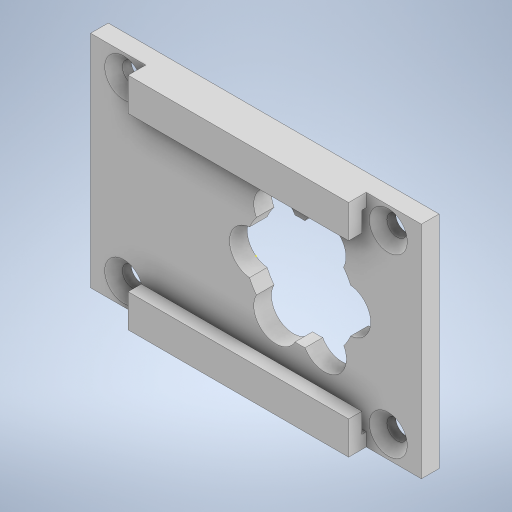
# Autodesk Inventor part: lid support
Saved by Autodesk Inventor 2023.3 (Build 273359000, 359)
## iProperties
Created: 2022-03-16
Part Number: lid support
Material: Generic
Document SubType Name: Modeling
Designer: sawtelles
Density: 1 g/cm^3
Appearance: Default
Author: sawtelles
Autodesk Inventor part; units mm, degrees
ref_plane "YZ Plane" through (0, 0, 0) normal (1, 0, 0) x (0, 1, 0)
ref_plane "XZ Plane" through (0, 0, 0) normal (0, 1, 0) x (-1, 0, 0)
ref_plane "XY Plane" through (0, 0, 0) normal (0, 0, 1) x (1, 0, 0)
sketch "Sketch1" plane through (0, 0, 0) normal (0, 0, 1) x (1, 0, 0)
  line L0 (37.5, -25) -> (-37.5, -25)
  line L1 (-37.5, -25) -> (-37.5, 25)
  line L2 (-37.5, 25) -> (37.5, 25)
  line L3 (37.5, 25) -> (37.5, -25)
  line L4 (37.5, -25) -> (-37.5, 25) construction
  line L5 (-37.5, -25) -> (37.5, 25) construction
  point P0 (0, 0)
  dimension "d0" = 75
  dimension "d1" = 50
  constraints: 12 end point, 2 midpoint, 2 parallel, 1 horizontal, 1 perpendicular
  measures "d0" distance of L1.end L2.end
  measures "d1" distance of L0.end L1.end
extrude "Extrusion1" add sketch "Sketch1" along normal blind 4
sketch "Sketch2" plane through (0, 0, 4) normal (0, 0, 1) x (1, 0, 0)
  point P0 (0, 0)
  point P1 (15.4, 10)
  point P2 (21, 0)
  point P3 (15.5, -10)
  point P4 (4.5, 10)
  point P5 (4.5, -10)
  point P6 (-1, 0)
hole "Hole1" at (15.4, 10, 4) at (21, 0, 4) at (15.5, -10, 4) at (4.5, 10, 4) at (4.5, -10, 4) at (-1, 0, 4) direction (0, 0, -1) diameter 10 end through all
sketch "Sketch3" plane through (0, 0, 4) normal (0, 0, 1) x (1, 0, 0)
  circle A0 centre (10, 0) radius 12.5
  line L0 (37.5, -25) -> (37.5, 25) projected
  point P0 (0, 0)
  dimension "d11" = 25
  dimension "d24" = 27.5
  constraints: 1 centre point
  measures "d11" diameter of A0
  measures "d24" distance from line of L0 A0.centre
extrude "Extrusion2" cut sketch "Sketch3" against normal blind 10
sketch "Sketch4" plane through (0, 0, 4) normal (0, 0, 1) x (1, 0, 0)
  point P0 (0, 0)
  point P1 (30, 20)
  point P2 (30, -20)
  point P3 (-30, 20)
  point P4 (-30, -20)
hole "Hole2" at (30, 20, 4) at (30, -20, 4) at (-30, 20, 4) at (-30, -20, 4) direction (0, 0, -1) diameter 4.6 end through all
chamfer "Chamfer1" distance 2 angle 45 4 edges at (-30, -17.7, 4) (30, -17.7, 4) (-30, 22.3, 4) (30, 22.3, 4)
sketch "Sketch5" plane through (0, 0, 4) normal (0, 0, 1) x (1, 0, 0)
  point P0 (0, 0)
sketch "Sketch6" plane through (0, 0, 4) normal (0, 0, 1) x (1, 0, 0)
  line L0 (37.5, 25) -> (-37.5, 25) projected
  line L1 (-25, 25) -> (25, 25)
  line L2 (25, 25) -> (25, 22)
  line L3 (25, 22) -> (-25, 22)
  line L4 (-25, 22) -> (-25, 25)
  line L5 (-37.5, -25) -> (37.5, -25) projected
  line L6 (-25, -25) -> (25, -25)
  line L7 (25, -25) -> (25, -22)
  line L8 (25, -22) -> (-25, -22)
  line L9 (-25, -22) -> (-25, -25)
  point P0 (0, 0)
  dimension "d25" = 50
  dimension "d26" = 3
  dimension "d27" = 3
  constraints: 16 end point, 4 parallel, 4 point on line, 2 horizontal, 2 perpendicular
  measures "d25" distance of L2.end L3.end
  measures "d26" distance of L1.end L2.end
  measures "d27" distance of L7.end L6.end
extrude "Extrusion3" add sketch "Sketch6" along normal blind 1
sketch "Sketch7" plane through (0, 0, 5) normal (0, 0, 1) x (1, 0, 0)
  line L0 (-25, 25) -> (-25, 22) projected
  line L1 (-25, 25) -> (25, 25)
  line L2 (25, 25) -> (25, 17.5)
  line L3 (25, 17.5) -> (-25, 17.5)
  line L4 (-25, 17.5) -> (-25, 25)
  line L5 (-37.5, -25) -> (37.5, -25) projected
  line L6 (-25, -25) -> (25, -25)
  line L7 (25, -25) -> (25, -17.5)
  line L8 (25, -17.5) -> (-25, -17.5)
  line L9 (-25, -17.5) -> (-25, -25)
  point P0 (0, 0)
  dimension "d30" = 50
  dimension "d31" = 7.5
  dimension "d32" = 7.5
  constraints: 16 end point, 4 parallel, 3 point on line, 2 horizontal, 2 perpendicular
  measures "d30" distance of L2.end L3.end
  measures "d31" distance of L1.end L2.end
  measures "d32" distance of L7.end L6.end
extrude "Extrusion4" add sketch "Sketch7" along normal blind 3
body "Solid1"
